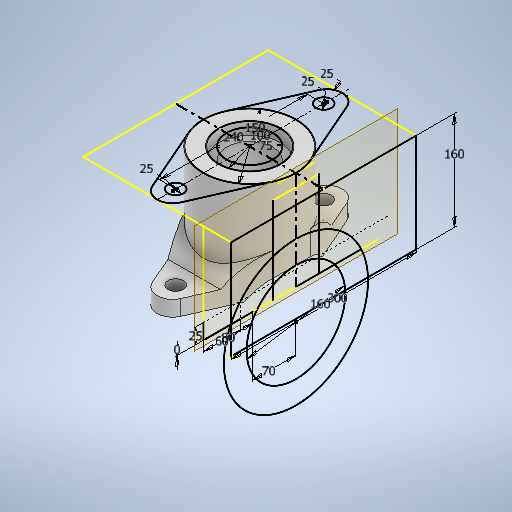
# Autodesk Inventor part: Baitap4
Saved by Autodesk Inventor 2025.2 (Build 292293000, 293)
## iProperties
Created: 2024-12-04
Part Number: Baitap4
Material: Generic
Document SubType Name: Modeling
Designer: hongquan
Density: 1 g/cm^3
Appearance: Default
Author: hongquan
Autodesk Inventor part; units mm, degrees
ref_plane "XZ Plane" through (0, 0, 0) normal (0, 1, 0) x (-1, 0, 0)
ref_plane "XY Plane" through (0, 0, 0) normal (0, 0, 1) x (1, 0, 0)
sketch "Sketch1" plane through (0, 0, 0) normal (1, 0, 0) x (0, 1, 0)
  point P0 (0, 0)
sketch "Sketch2" plane through (0, 0, 0) normal (1, 0, 0) x (0, 1, 0)
  line L0 (0, 0) -> (160, 0)
  line L1 (160, 0) -> (160, -300)
  line L2 (160, -300) -> (0, -300)
  line L3 (0, -300) -> (0, 0)
  dimension "d0" = 300
  dimension "d1" = 160
  constraints: 8 end point, 2 parallel, 1 horizontal, 1 perpendicular
  measures "d0" distance of L2.end L0.start
  measures "d1" distance of L1.end L2.end
extrude "Extrusion1" add sketch "Sketch2" against normal blind 240
sketch "Sketch3" plane through (0, 160, 0) normal (0, 1, 0) x (1, 0, 0)
  line L0 (-240, 300) -> (-240, 0) projected
  line L1 (-240, 150) -> (0, 150)
  line L2 (0, 0) -> (0, 300) projected
  line L3 (0, 0) -> (-240, 0) projected
  line L4 (-120, 0) -> (-120, 300) construction
  circle A0 centre (-120, 150) radius 75
  circle A1 centre (-120, 150) radius 50
  circle A2 centre (-120, 150) radius 37.5
  line L5 (-120, 30) -> (-120, 270) construction
  circle A3 centre (-120, 270) radius 12.5
  circle A4 centre (-120, 30) radius 12.5
  line L6 (0, 300) -> (-240, 300) projected
  line L7 (-188.7386, 180) -> (-142.9129, 285)
  line L8 (-51.2614, 180) -> (-97.0871, 285)
  arc A5 (-97.0871, 285) -> (-142.9129, 285) centre (-120, 275) ccw
  line L9 (-188.7386, 120) -> (-142.9129, 15)
  line L10 (-51.2614, 120) -> (-97.0871, 15)
  arc A6 (-142.9129, 15) -> (-97.0871, 15) centre (-120, 25) ccw
  point P0 (-120, 300)
  point P1 (-120, 300)
  point P2 (-120, 0)
  dimension "d4" = 150
  dimension "d5" = 100
  dimension "d6" = 75
  dimension "d7" = 240
  dimension "d8" = 25
  dimension "d9" = 25
  dimension "d13" = 25
  constraints: 14 end point, 7 midpoint, 7 symmetric about line, 6 centre point, 4 coincident, 4 point on circle, 2 vertical, 1 point on line, 1 tangent, 6 other
  measures "d5" diameter of A1
  measures "d6" diameter of A2
  measures "d7" distance of L5.start L5.end
  measures "d8" diameter of A3
  measures "d9" diameter of A4
  measures "d13" radius of A5
extrude "Extrusion2" cut sketch "Sketch3" against normal blind 160 contours L6 A5 L7 A0 L1 L0 | L1 A0 L9 A6 L3 L0 | L6 L2 L1 A0 L8 A5 | A6 L10 A0 L1 L2 L3
extrude "Extrusion3" cut sketch "Sketch3" against normal blind 160 contours A3 | A4
extrude "Extrusion4" cut sketch "Sketch3" against normal blind 160 contours A2 L1 | L1 A2
extrude "Extrusion5" cut sketch "Sketch3" against normal blind 20 contours A1 L1 A2 | L1 A2 A1
ref_plane "Work Plane1" through (-45, 160, -150) normal (1, 0, 0) x (0, 1, 0)
sketch "Sketch4" plane through (-45, 160, -150) normal (1, 0, 0) x (0, 1, 0)
  circle A0 centre (-209.6065, 0) radius 80
  line L0 (-20, -37.5) -> (-160, -37.5) projected
  line L1 (-160, -37.5) -> (-160, 37.5) projected
  line L2 (-20, -37.5) -> (-160, -37.5)
  line L3 (-20, -37.5) -> (-20, 37.5) projected
  line L4 (-20, 37.5) -> (-160, 37.5)
  line L5 (-160, 135) -> (-160, 30) projected
  line L6 (0, -30) -> (0, 30) projected
  line L7 (0, 0) -> (-160, 0)
  line L8 (-160, 150) -> (-160, 70)
  line L9 (-160, 150) -> (-160, 90)
  line L10 (-160, 150) -> (-135, 150)
  line L11 (-160, 150) -> (0, 150) projected
  line L12 (-135, 150) -> (-135, -149.8181) construction
  line L13 (-160, 90) -> (-135, 90) construction
  circle A1 centre (-209.6065, 0) radius 116.9023
  line L14 (-160, 105.8552) -> (-160, 62.763) construction
  line L15 (-160, -62.763) -> (-160, -105.8552) construction
  line L16 (-160, 0) -> (-160, -105.8552)
  line L17 (-160, -132.5) -> (-160, -107.5) projected
  point P0 (-160, -62.763)
  point P1 (-160, 105.8552)
  dimension "d22" = 160
  dimension "d23" = 80
  dimension "d24" = 0
  dimension "d25" = 70
  dimension "d26" = 60
  dimension "d31" = 25
  constraints: 22 end point, 7 point on line, 5 point on circle, 3 perpendicular, 2 centre point, 2 coincident, 2 midpoint, 2 vertical, 1 collinear, 1 horizontal, 1 other
  measures "d22" diameter of A0
  measures "d23" distance of L8.start L8.end
  measures "d24" distance between parallel lines of L5 L8
  measures "d25" vertical distance of A0.centre L8.end
  measures "d26" distance of L9.start L9.end
  measures "d31" distance of L9.start L10.end
extrude "Extrusion6" cut sketch "Sketch4" against normal blind 150 contours L7 L1 L4 A0 | A0 L0 L1 L7 | L4 L5 A0 | A0 L16 L0 | L1 L16 A0 L5
extrude "Extrusion7" cut sketch "Sketch3" against normal blind 135 contours A5 L8 A0 L7 | A6 L9 A0 L10
extrude "Extrusion8" add sketch "Sketch4" against normal blind 135 contours L7 A1 L0 A0 | A0 L4 A1 L7 | A0 L5 A1 L4 | L0 A1 L16 A0 | A0 L16 A1 L5
extrude "Extrusion9" cut sketch "Sketch4" against normal blind 135 contours A0 L16 A1 L5
extrude "Extrusion10" cut sketch "Sketch3" against normal blind 200 contours L6 A5 L7 A0 L1 L0 | L1 A0 L9 A6 L3 L0 | L6 L2 L1 A0 L8 A5 | A6 L10 A0 L1 L2 L3
body "Solid1"
